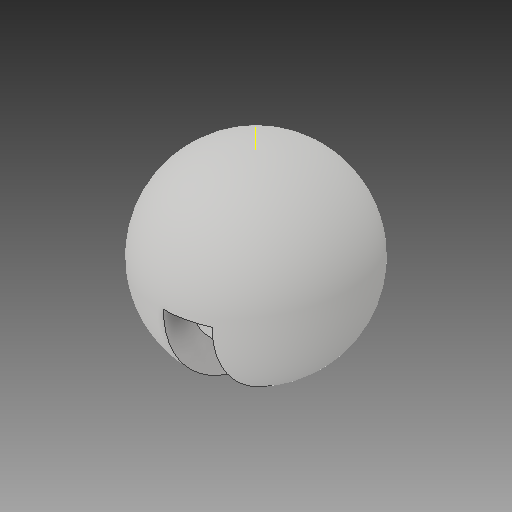
# Autodesk Inventor part: ДЗ 3 Курганова
Saved by Autodesk Inventor 2017 (Build 210142000, 142)
## iProperties
Created: 2017-03-29
Part Number: ДЗ 3 Курганова
Material: Типовые
Document SubType Name: Modeling
Designer: Student
Density: 1 g/cm^3
Appearance: По умолчанию
Mass: 100.007 g
Surface Area: 226.2 cm^2
Volume: 100.007 cm^3
Author: Student
Autodesk Inventor part; units mm, degrees
ref_plane "YZ Plane" through (0, 0, 0) normal (1, 0, 0) x (0, 1, 0)
ref_plane "XZ Plane" through (0, 0, 0) normal (0, 1, 0) x (-1, 0, 0)
ref_plane "XY Plane" through (0, 0, 0) normal (0, 0, 1) x (1, 0, 0)
sketch "Эскиз1" plane through (0, 0, 0) normal (0, 0, 1) x (1, 0, 0)
  arc A0 (0, -35) -> (0, 35) centre (0, 0) ccw
  arc A1 (0, -25) -> (0, 25) centre (0, 0) ccw
  line L0 (0, 35) -> (0, 25)
  line L1 (0, -25) -> (0, -35)
  line L2 (0, -49) -> (0, 49) projected
  dimension "d0" = 25
  dimension "d1" = 35
  dimension "d2" = 10
  dimension "d3" = 10
  constraints: 5 point on circle, 4 end point, 2 centre point, 2 coincident, 1 collinear, 1 vertical
  measures "d0" radius of A1
  measures "d1" radius of A0
  measures "d2" distance of L0.start L0.end
  measures "d3" distance of L1.start L1.end
revolve "Вращение1" add sketch "Эскиз1" angle 360 about axis through (0, -10, 0) along (0, 1, 0) contours L1 A1 L0 A0
sketch "Эскиз2" plane through (0, 0, 0) normal (0, 0, 1) x (1, 0, 0)
  line L0 (0, 0) -> (15, 0)
  line L1 (15, 0) -> (15, -48.4615)
  line L2 (0, -48.4615) -> (0, 0)
  dimension "d5" = 15
  constraints: 6 end point, 1 horizontal, 1 parallel, 1 perpendicular
  measures "d5" distance of L2.start L1.end
extrude "Выдавливание1" cut sketch "Эскиз2" along normal through all both and the other way through all fills toward (0.05, -24.2308) open curves L2 L0 L1
